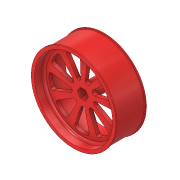
# Autodesk Inventor part: Custom Wheel
Saved by Autodesk Inventor 2019.4 (Build 234330000, 330)
## iProperties
Created: 2020-01-04
Part Number: Custom Wheel
Material: Aluminum 6061
Document SubType Name: Modeling
Designer: mavericks
Density: 2.7 g/cm^3
Appearance: Aluminum - Flat
Mass: 202.572 g
Surface Area: 460.844 cm^2
Volume: 75.0267 cm^3
Author: mavericks
Autodesk Inventor part; units mm, degrees
ref_plane "YZ Plane" through (0, 0, 0) normal (1, 0, 0) x (0, 1, 0)
ref_plane "XZ Plane" through (0, 0, 0) normal (0, 1, 0) x (-1, 0, 0)
sketch "Sketch1" plane through (0, 0, 0) normal (0, 0, 1) x (1, 0, 0)
  circle A0 centre (0, 0) radius 55.88
  circle A1 centre (0, 0) radius 9.525
  line L0 (7.391, 0) -> (3.6955, -6.4008)
  line L1 (3.6955, -6.4008) -> (-3.6955, -6.4008)
  line L2 (-3.6955, -6.4008) -> (-7.391, 0)
  line L3 (-7.391, 0) -> (-3.6955, 6.4008)
  line L4 (-3.6955, 6.4008) -> (3.6955, 6.4008)
  line L5 (3.6955, 6.4008) -> (7.391, 0)
  circle A2 centre (0, 0) radius 52.705
  point P0 (0, 9.525)
  dimension "d1" = 19.05
  dimension "d0" = 111.76
  dimension "d2" = 12.8016
  dimension "d3" = 3.175
  constraints: 12 end point, 3 coincident, 2 centre point, 1 horizontal alignment, 1 vertical alignment, 15 other
  measures "d0" diameter of A0
  measures "d2" distance between parallel lines of L1 L4
  measures "d3" radial gap between concentric circles of A0 A2
extrude "Extrusion1" add sketch "Sketch1" along normal mid plane 41.275 contours A0 | A1 | A2
sketch "Sketch4" plane through (0, 0, 20.6375) normal (0, 0, 1) x (1, 0, 0)
  circle A0 centre (0, 0) radius 52.705
  circle A1 centre (0, 0) radius 55.88 construction
  dimension "d59" = 3.175
  constraints: 1 centre point, 1 coincident
  measures "d59" radial gap between concentric circles of A0 A1
extrude "Extrusion4" cut sketch "Sketch4" against normal blind 12.7
sketch "Sketch5" plane through (0, 0, -20.6375) normal (0, 0, -1) x (-1, 0, 0)
  circle A0 centre (0, 0) radius 9.525
  line L0 (3.6955, 6.4008) -> (7.391, 0) projected
  line L1 (7.391, 0) -> (3.6955, -6.4008)
  line L2 (3.6955, -6.4008) -> (-3.6955, -6.4008)
  line L3 (-3.6955, -6.4008) -> (-7.391, 0)
  line L4 (-7.391, 0) -> (-3.6955, 6.4008)
  line L5 (-3.6955, 6.4008) -> (3.6955, 6.4008)
  line L6 (3.6955, 6.4008) -> (7.391, 0)
  dimension "d26" = 19.05
  constraints: 12 end point, 2 coincident, 1 centre point, 13 other
  measures "d26" diameter of A0
extrude "Extrusion5" add sketch "Sketch5" along normal blind 3.175
sketch "Sketch6" plane through (0, 0, -20.6375) normal (0, 0, -1) x (-1, 0, 0)
  circle A0 centre (0, 0) radius 52.705
  circle A1 centre (0, 0) radius 9.525
  circle A2 centre (0, 0) radius 55.88 construction
  dimension "d60" = 3.175
  constraints: 2 centre point, 2 coincident
  measures "d60" radial gap between concentric circles of A0 A2
extrude "Extrusion6" cut sketch "Sketch6" against normal blind 23.8252
sketch "Sketch7" plane through (0, 0, 7.9375) normal (0, 0, 1) x (1, 0, 0)
  circle A0 centre (0, 0) radius 9.525 projected
  circle A1 centre (0, 0) radius 52.705 projected
  circle A2 centre (0, 0) radius 47.9425 construction
  circle A3 centre (0, 0) radius 14.2875 construction
  line L0 (-9.7714, 10.4237) -> (-9.7714, 46.9362) construction
  line L1 (-9.7714, 10.4237) -> (16.8454, 44.8856)
  line L2 (-9.7714, 10.4237) -> (-36.3881, 44.8856)
  arc A4 (16.8454, 44.8856) -> (-36.3881, 44.8856) centre (-9.7714, -126.8345) ccw
  point P0 (-6.5143, 6.9491)
  dimension "d42" = 4.7625
  dimension "d41" = 4.7625
  dimension "d43" = 34.4619
  dimension "d44" = 36.5125
  dimension "d45" = 4.7625
  constraints: 6 end point, 5 point on circle, 2 centre point, 1 symmetric about line, 1 vertical, 5 other
  measures "d41" radial gap between concentric circles of A1 A2
  measures "d43" vertical distance of L0.start L1.end
  measures "d44" distance of L0.start L0.end
  measures "d45" distance of point (-6.514, 6.949) L0.start
extrude "Extrusion8" [suppressed]
fillet "Fillet1" [suppressed]
pattern_circular "Circular Pattern1" [suppressed]
fillet "Fillet2" [suppressed]
sketch "Sketch8" plane through (0, 0, 20.6375) normal (0, 0, 1) x (1, 0, 0)
  circle A0 centre (0, 0) radius 55.88 projected
  circle A1 centre (0, 0) radius 57.15
  dimension "d53" = 114.3
  constraints: 1 centre point, 1 coincident
  measures "d53" diameter of A1
extrude "Extrusion9" add sketch "Sketch8" against normal blind 1.5875
ref_plane "Work Plane1" through (0, 0, 0) normal (0, 0, 1) x (1, 0, 0)
mirror "Mirror1" about plane through (0, 0, 0) normal (0, 0, 1) of "Extrusion9"
fillet "Fillet3" radius 3.175 1 edges at (9.525, 0, 3.1877)
fillet "Fillet4" radius 3.175 1 edges at (-52.705, 0, 7.9375)
fillet "Fillet5" radius 3.175 1 edges at (52.705, 0, 3.1877)
sketch "Sketch9" plane through (0, 0, 3.1877) normal (0, 0, -1) x (-1, 0, 0)
  circle A0 centre (0, 0) radius 12.7 construction
  circle A1 centre (0, 0) radius 49.53 construction
  circle A2 centre (0, 0) radius 12.7 construction
  line L0 (0, -12.7) -> (0, -17.78) construction
  arc A3 (3.0152, -16.7853) -> (-3.1007, -17.0973) centre (0, -17.78) ccw
  circle A4 centre (0, 0) radius 49.53 construction
  line L1 (3.0152, -16.7853) -> (10.9727, -40.9066)
  line L2 (-3.1007, -17.0973) -> (-8.5623, -41.9032)
  arc A5 (8.941, -44.8445) -> (10.9502, -40.8384) centre (7.935, -41.8331) ccw
  arc A6 (-8.4774, -41.5179) -> (-6.215, -45.2629) centre (-5.3767, -42.2006) ccw
  arc A7 (-6.215, -45.2629) -> (8.941, -44.8445) centre (0.674, -20.0971) ccw
  point P0 (-10.4488, -48.4153)
  point P1 (10.4488, -48.4153)
  dimension "d62" = 5.08
  dimension "d63" = 6.35
  dimension "d77" = 25.4
  dimension "d78" = 25.4
  dimension "d79" = 6.35
  dimension "d80" = 6.35
  dimension "d81" = 13.3117
  dimension "d82" = 24.0531
  dimension "d83" = 42.2006
  dimension "d84" = 26.0917
  dimension "d85" = 17.78
  constraints: 10 point on circle, 6 end point, 6 tangent, 4 centre point, 2 point on line, 1 coincident, 1 vertical, 1 vertical alignment, 1 other
  measures "d62" distance of L0.start L0.end
  measures "d63" diameter of A3
  measures "d77" distance of L1.start L1.end
  measures "d78" distance of L2.start L2.end
  measures "d79" diameter of A5
  measures "d80" diameter of A6
  measures "d81" horizontal distance of A6.centre A5.centre
  measures "d82" vertical distance of A5.centre L0.end
  measures "d83" vertical distance of A1.centre A6.centre
  measures "d84" radius of A7
  measures "d85" distance of A1.centre L0.end
extrude "Extrusion10" cut sketch "Sketch9" against normal up to next
pattern_circular "Circular Pattern2" count 9 over 360 about axis through (0, 0, -20.6375) along (0, 0, -1) of "Extrusion10"
body "Solid1"
